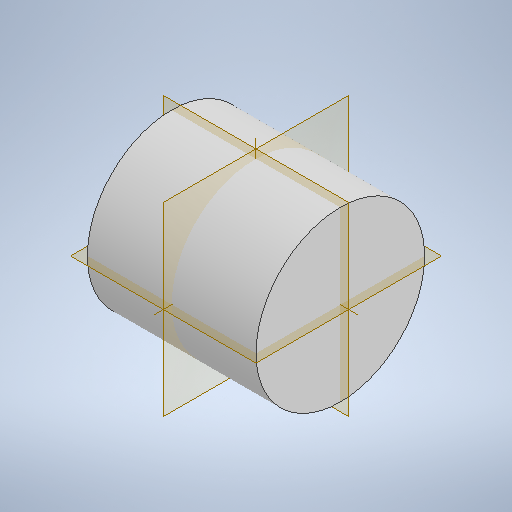
# Autodesk Inventor part: peca_011_001
Saved by Autodesk Inventor 2026 (Build 300175000, 175)
## iProperties
Created: 2025-03-26
Part Number: peca_011_001
Material: Generic
Document SubType Name: Modeling
Designer: Carlos Dias
Density: 1 g/cm^3
Appearance: Default
Author: Carlos Dias
Autodesk Inventor part; units mm, degrees
sketch "Sketch1" plane through (0, 0, 0) normal (1, 0, 0) x (0, 1, 0)
  circle A0 centre (0, 0) radius 2.5
  dimension "d0" = 5
  constraints: 1 centre point, 1 coincident
  measures "d0" diameter of A0
extrude "Extrusion1" add sketch "Sketch1" along normal mid plane 5
body "Solid1"
